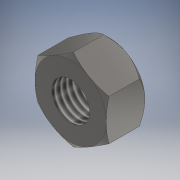
# Autodesk Inventor part: AxleNut
Saved by Autodesk Inventor 2019 (Build 230136000, 136)
## iProperties
Created: 2020-12-09
Part Number: AxleNut
Material: Steel, Carbon
Document SubType Name: Modeling
Designer: Anass Hamdi
Density: 7.85 g/cm^3
Appearance: Semi-Polished
Author: Anass Hamdi
Autodesk Inventor part; units mm, degrees
ref_plane "YZ Plane" through (0, 0, 0) normal (1, 0, 0) x (0, 1, 0)
sketch "Sketch1" plane through (0, 0, 0) normal (0, 0, 1) x (1, 0, 0)
  line L0 (0, 7.3323) -> (6.35, 3.6662)
  line L1 (6.35, 3.6662) -> (6.35, -3.6662)
  line L2 (6.35, -3.6662) -> (0, -7.3323)
  line L3 (0, -7.3323) -> (-6.35, -3.6662)
  line L4 (-6.35, -3.6662) -> (-6.35, 3.6662)
  line L5 (-6.35, 3.6662) -> (0, 7.3323)
  point P0 (0, 0)
  point P1 (0, 0)
  dimension "d1" = 12.7
  constraints: 12 end point, 1 coincident, 13 other
  measures "d1" distance between parallel lines of L1 L4
extrude "Extrusion1" add sketch "Sketch1" along normal mid plane 6.9
sketch "Sketch2" plane through (0, 0, -3.45) normal (0, 0, -1) x (-1, 0, 0)
  line L0 (3.175, 5.4993) -> (6.35, 3.6662)
  line L1 (6.35, 3.6662) -> (6.35, 0)
  arc A0 (6.35, 0) -> (3.175, 5.4993) centre (0, 0) ccw
  constraints: 4 end point, 2 point on circle, 1 centre point
ref_plane "Work Plane1" through (0, 0, -2.45) normal (0, 0, -1) x (-1, 0, 0)
sketch "Sketch3" plane through (0, 0, -2.45) normal (0, 0, -1) x (-1, 0, 0)
  line L0 (3.9625, 6.1695) -> (7.5244, 3.8817)
  line L1 (7.5244, 3.8817) -> (7.3241, -0.3469)
  arc A0 (7.3241, -0.3469) -> (3.9625, 6.1695) centre (0, 0) ccw
  constraints: 4 end point, 2 point on circle, 1 centre point, 1 tangent
loft "Loft1" cut profiles "Sketch2", "Sketch3"
pattern_circular "Circular Pattern1" count 6 over 360 about axis through (0, 0, -10) along (0, 0, 1) of "Loft1"
ref_plane "Work Plane2" through (0, 0, 2.95) normal (0, 0, 1) x (1, 0, 0)
sketch "Sketch4" plane through (0, 0, 3.45) normal (0, 0, 1) x (1, 0, 0)
  line L0 (-3.175, -5.4993) -> (-6.35, -3.6662)
  line L1 (-6.35, -3.6662) -> (-6.35, 0)
  arc A0 (-6.35, 0) -> (-3.175, -5.4993) centre (0, 0) ccw
  constraints: 4 end point, 2 point on circle, 1 centre point
sketch "Sketch5" plane through (0, 0, 2.95) normal (0, 0, 1) x (1, 0, 0)
  line L0 (-3.6816, -6.3411) -> (-7.3426, -4.2155)
  line L1 (-7.3426, -4.2155) -> (-7.3323, 0.0178)
  arc A0 (-7.3323, 0.0178) -> (-3.6816, -6.3411) centre (0, 0) ccw
  constraints: 4 end point, 2 point on circle, 1 centre point, 1 tangent
loft "Loft2" cut profiles "Sketch4", "Sketch5"
pattern_circular "Circular Pattern2" count 6 over 360 about axis through (0, 0, -10) along (0, 0, 1) of "Loft2"
sketch "Sketch6" plane through (0, 0, -3.45) normal (0, 0, -1) x (-1, 0, 0)
  point P0 (0, 0)
  point P1 (0, 0)
  constraints: 1 coincident
hole "Hole1" at (0, 0, -3.45) direction (0, 0, 1) diameter 6.782 depth 6.9 thread size "5/16-24 UNF" class "2B" standard "ANSI Unified Screw Threads"
body "Solid1"
